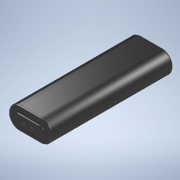
# Autodesk Inventor part: onxp5510
Saved by Autodesk Inventor 2020.2 (Build 242310000, 310)
## iProperties
Created: 2019-11-09
Part Number: onxp5510
Material: Silicon Nitride
Document SubType Name: Modeling
Designer: agmle
Density: 3.18 g/cm^3
Appearance: Glossy - Black
Mass: 459.912 g
Surface Area: 190.28 cm^2
Volume: 144.626 cm^3
Author: agmle
Autodesk Inventor part; units mm, degrees
ref_plane "YZ Plane" through (0, 0, 0) normal (1, 0, 0) x (0, 1, 0)
ref_plane "XZ Plane" through (0, 0, 0) normal (0, 1, 0) x (-1, 0, 0)
ref_plane "XY Plane" through (0, 0, 0) normal (0, 0, 1) x (1, 0, 0)
sketch "Sketch1" plane through (0, 0, 0) normal (0, 0, 1) x (1, 0, 0)
  arc A0 (-11.684, 12.319) -> (-11.684, -12.319) centre (-11.684, 0) ccw
  arc A1 (11.684, -12.319) -> (11.684, 12.319) centre (11.684, 0) ccw
  line L0 (-11.684, 12.319) -> (11.684, 12.319)
  line L1 (11.684, -12.319) -> (-11.684, -12.319)
  line L2 (-11.684, 0) -> (11.684, 0) construction
  line L3 (-11.684, 0) -> (-24.003, 0) construction
  line L4 (11.684, 0) -> (24.003, 0) construction
  point P0 (0, 0)
  point P1 (0, 0)
  dimension "d0" = 24.638
  dimension "d1" = 48.006
  constraints: 10 end point, 6 point on circle, 3 tangent, 2 centre point, 2 horizontal, 1 coincident, 1 equal radius, 1 midpoint, 1 parallel
  measures "d0" distance between parallel lines of L1 L0
  measures "d1" distance of L4.end L3.end
extrude "Extrusion1" add sketch "Sketch1" along normal blind 136.906
sketch "Sketch2" plane through (0, 0, 136.906) normal (0, 0, 1) x (1, 0, 0)
  arc A0 (-11.303, 5.842) -> (-11.303, -5.842) centre (-11.303, 0) ccw
  arc A1 (11.303, -5.842) -> (11.303, 5.842) centre (11.303, 0) ccw
  line L0 (-11.303, 5.842) -> (11.303, 5.842)
  line L1 (11.303, -5.842) -> (-11.303, -5.842)
  line L2 (-17.145, 0) -> (17.145, 0) construction
  point P0 (0, 0)
  point P1 (0, 0)
  dimension "d4" = 34.29
  dimension "d5" = 11.684
  constraints: 6 end point, 6 point on circle, 4 tangent, 2 centre point, 2 point on line, 1 coincident, 1 equal radius, 1 horizontal, 1 midpoint
  measures "d4" distance of L2.end L2.start
  measures "d5" distance between parallel lines of L1 L0
extrude "Extrusion2" add sketch "Sketch2" along normal blind 1.905
fillet "Fillet1" radius 1.5875 12 edges at (-24.003, 0, 136.906) (0, -12.319, 136.906) (24.003, 0, 136.906) (0, 12.319, 136.906) (-24.003, 0, 0) (0, -12.319, 0) (24.003, 0, 0) (0, 12.319, 0) (-17.145, 0, 138.811) (0, -5.842, 138.811) (17.145, 0, 138.811) (0, 5.842, 138.811)
sketch "Sketch3" plane through (0, 0, 138.811) normal (0, 0, 1) x (1, 0, 0)
  line L0 (-4.318, 0) -> (4.318, 0) construction
  point P0 (0, 0)
  point P1 (0, 0)
  dimension "d9" = 8.636
  constraints: 2 end point, 1 coincident, 1 horizontal, 1 midpoint
  measures "d9" distance of L0.start L0.end
body "Solid1"
